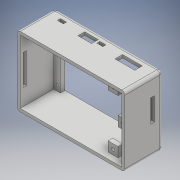
# Autodesk Inventor part: ttgofront
Saved by Autodesk Inventor 2017 (Build 210142000, 142)
## iProperties
Created: 2018-11-11
Part Number: ttgofront
Material: Generic
Document SubType Name: Modeling
Designer: simulator
Density: 1 g/cm^3
Appearance: Default
Author: simulator
Autodesk Inventor part; units mm, degrees
ref_plane "YZ Plane" through (0, 0, 0) normal (1, 0, 0) x (0, 1, 0)
ref_plane "XZ Plane" through (0, 0, 0) normal (0, 1, 0) x (-1, 0, 0)
ref_plane "XY Plane" through (0, 0, 0) normal (0, 0, 1) x (1, 0, 0)
sketch "Sketch1" plane through (0, 0, 0) normal (0, 1, 0) x (-1, 0, 0)
  line L0 (0, 21) -> (-67, 21)
  line L1 (-67, 21) -> (-67, -21)
  line L2 (-67, -21) -> (0, -21)
  line L3 (0, -21) -> (0, 21)
  line L4 (-4.5, 21) -> (-4.5, -21)
  line L5 (-60.5, 21) -> (-60.5, -21)
  line L6 (2, 23) -> (-69, 23)
  line L7 (-69, 23) -> (-69, -23)
  line L8 (-69, -23) -> (2, -23)
  line L9 (2, -23) -> (2, 23)
  line L10 (-32.322, -31.2235) -> (-36.822, -31.2235)
  line L11 (-36.822, -31.2235) -> (-36.822, -37.7235)
  line L12 (-36.822, -37.7235) -> (-32.322, -37.7235)
  line L13 (-32.322, -37.7235) -> (-32.322, -31.2235)
  line L14 (-32.322, -37.7235) -> (-36.822, -31.2235)
  line L15 (-67, -8.75) -> (-67, -15.25)
  line L16 (-67, 2.25) -> (-67, -4.25)
  line L17 (-67, 12.25) -> (-67, 5.75)
  line L18 (-66, -15.25) -> (-61.5, -15.25)
  line L19 (-61.5, -15.25) -> (-61.5, 14.25)
  line L20 (-61.5, 14.25) -> (-66, 14.25)
  line L21 (-66, 14.25) -> (-66, -15.25)
  point P0 (0, 0)
  point P1 (0, 0)
  point P2 (-2.5, -17.5)
  point P3 (-2.5, 18.5)
  point P4 (-63.5, 18.5)
  point P5 (-63.5, -17.5)
  point P6 (-34.572, -34.4735)
  dimension "d0" = 67
  dimension "d1" = 42
  dimension "d5" = 2.5
  dimension "d6" = 36
  dimension "d7" = 2.5
  dimension "d8" = 3.5
  dimension "d9" = 2.5
  dimension "d10" = 3.5
  dimension "d11" = 3.5
  dimension "d12" = 4.5
  dimension "d13" = 6.5
  dimension "d14" = 2
  dimension "d20" = 4.5
  dimension "d21" = 6.5
  dimension "d97" = 6.5
  dimension "d99" = 6.5
  dimension "d107" = 6.5
  dimension "d108" = 1
  dimension "d111" = 6.75
  dimension "d112" = 5.75
  dimension "d113" = 4.5
  constraints: 44 end point, 8 parallel, 6 perpendicular, 4 point on line, 3 horizontal, 2 midpoint, 1 coincident, 3 other
  measures "d0" distance of L2.end L1.end
  measures "d1" distance of L2.end L0.start
  measures "d5" distance from line of point (-2.5, -17.5) L3
  measures "d6" distance of point (-2.5, -17.5) point (-2.5, 18.5)
  measures "d7" distance from line of L0 point (-2.5, 18.5)
  measures "d8" distance from line of point (-63.5, 18.5) L1
  measures "d9" distance from line of L0 point (-63.5, 18.5)
  measures "d10" distance from line of point (-63.5, -17.5) L1
  measures "d11" distance from line of point (-63.5, -17.5) L2
  measures "d12" distance between parallel lines of L3 L4
  measures "d13" distance between parallel lines of L5 L1
  measures "d14" distance between parallel lines of L6 L0
  measures "d20" distance of L12.end L11.end
  measures "d21" distance of L11.end L10.end
  measures "d97" distance of L15.end L15.start
  measures "d99" distance of L16.end L16.start
  measures "d107" distance of L17.end L17.start
  measures "d108" distance from line of L18.start L1
  measures "d111" distance between parallel lines of L0 L20
  measures "d112" distance between parallel lines of L2 L18
  measures "d113" distance of L19.end L20.end
extrude "Extrusion1" add sketch "Sketch1" along normal blind 3 contours L3 L2 L4 L0 | L5 L2 L1 L0 | L9 L8 L7 L6 | L21 L20 L19 L18
sketch "Sketch2" plane through (0, 0, 0) normal (0, -1, 0) x (1, 0, 0)
  point P0 (0, 0)
  point P1 (2.5, 18.5)
  point P2 (2.5, -17.5)
  point P3 (63.5, -17.5)
  point P4 (63.5, 18.5)
hole "Hole1" at (2.5, 0, -17.5) at (2.5, 0, 18.5) at (63.5, 0, 18.5) at (63.5, 0, -17.5) direction (0, 1, 0) diameter 1.5 depth 2 tip angle 118
extrude "Extrusion2" add sketch "Sketch1" against normal blind 15 contours L9 L8 L7 L6
fillet "Fillet1" radius 2 8 edges at (-2, -6, 23) (-2, -6, -23) (69, -6, 23) (69, -6, -23) (33.5, 3, -23) (69, 3, 0) (33.5, 3, 23) (-2, 3, 0)
sketch "Sketch3" plane through (-2, -15, -21) normal (-1, 0, 0) x (0, 0, 1)
  line L0 (42, 15) -> (0, 15) projected
  line L1 (42, 16) -> (42, 0) projected
  point P0 (21, 15)
  point P1 (34.5, 7.5)
  dimension "d40" = 7.5
  dimension "d41" = 7.5
  measures "d40" distance from line of point (34.5, 7.5) L0
  measures "d41" distance from line of point (34.5, 7.5) L1
hole "Hole2" at (-2, -7.5, 13.5) direction (1, 0, 0) diameter 5.5 depth 5 tip angle 118
sketch "Sketch4" plane through (0, -15, 0) normal (0, -1, 0) x (1, 0, 0)
  arc A0 (67, -23) -> (69, -21) centre (67, -21) ccw projected
  line L0 (69, -21) -> (69, 21) projected
  arc A1 (69, 21) -> (67, 23) centre (67, 21) ccw projected
  line L1 (67, 23) -> (0, 23) projected
  arc A2 (0, 23) -> (-2, 21) centre (0, 21) ccw projected
  line L2 (-2, 21) -> (-2, -21) projected
  arc A3 (-2, -21) -> (0, -23) centre (0, -21) ccw projected
  line L3 (0, -23) -> (67, -23) projected
  line L4 (67, -21) -> (0, -21) projected
  line L5 (0, -21) -> (0, 21) projected
  line L6 (0, 21) -> (67, 21) projected
  line L7 (67, 21) -> (67, -21) projected
  line L8 (67, 21) -> (60.5, 21) projected
  line L9 (67, 21) -> (62, 21)
  line L10 (62, 21) -> (62, 16)
  line L11 (62, 16) -> (67, 16)
  line L12 (67, 16) -> (67, 21)
  line L13 (60.5, -21) -> (67, -21) projected
  line L14 (67, -21) -> (62, -21)
  line L15 (62, -21) -> (62, -16)
  line L16 (62, -16) -> (67, -16)
  line L17 (67, -16) -> (67, -21)
  line L18 (0, -21) -> (5, -21)
  line L19 (5, -21) -> (5, -16)
  line L20 (5, -16) -> (0, -16)
  line L21 (0, -16) -> (0, -21)
  line L22 (0, 21) -> (5, 21)
  line L23 (5, 21) -> (5, 16)
  line L24 (5, 16) -> (0, 16)
  line L25 (0, 16) -> (0, 21)
  point P0 (0, 0)
  dimension "d49" = 5
  dimension "d50" = 5
  dimension "d51" = 5
  dimension "d52" = 5
  dimension "d53" = 5
  dimension "d54" = 5
  dimension "d55" = 5
  dimension "d56" = 5
  constraints: 32 end point, 8 parallel, 4 horizontal, 4 perpendicular
  measures "d49" distance of L11.end L10.end
  measures "d50" distance of L10.end L9.end
  measures "d51" distance of L15.end L16.end
  measures "d52" distance of L14.end L15.end
  measures "d53" distance of L20.end L19.end
  measures "d54" distance of L19.end L18.end
  measures "d55" distance of L23.end L24.end
  measures "d56" distance of L22.end L23.end
sketch "Sketch6" plane through (69, 1, 21) normal (1, 0, 0) x (0, 0, -1)
  line L0 (42, 0) -> (42, -16) projected
  line L1 (0, 0) -> (42, 0) projected
  line L2 (0, -16) -> (0, 0) projected
  line L3 (42, -1) -> (0, -1) projected
  line L4 (25, -3.5) -> (10, -3.5)
  line L5 (10, -3.5) -> (10, -6)
  line L6 (10, -6) -> (25, -6)
  line L7 (25, -6) -> (25, -3.5)
  line L8 (42, -1) -> (42, -16) projected
  line L9 (0, -1) -> (0, -16) projected
  line L10 (42, -1) -> (0, -1) projected
  line L11 (0, -16) -> (42, -16) projected
  line L12 (42, -16) -> (0, -16) projected
  point P0 (21, -1)
  dimension "d68" = 15
  dimension "d69" = 2.5
  dimension "d70" = 10
  dimension "d71" = 2.5
  constraints: 8 end point, 2 parallel, 1 horizontal, 1 perpendicular
  measures "d68" distance of L6.end L5.end
  measures "d69" distance of L5.end L4.end
  measures "d70" distance between parallel lines of L5 L2
  measures "d71" distance between parallel lines of L3 L4
extrude "Extrusion5" cut sketch "Sketch6" against normal blind 10 contours L7 L6 L5 L4
sketch "Sketch7" plane through (0, 1, 23) normal (0, 0, 1) x (1, 0, 0)
  line L0 (67, 0) -> (67, 2) projected
  line L1 (67, 2) -> (60.5, 2) projected
  line L2 (60.5, 2) -> (4.5, 2) projected
  line L3 (4.5, 2) -> (0, 2) projected
  line L4 (0, 2) -> (0, 0) projected
  line L5 (0, 0) -> (67, 0) projected
  line L6 (67, 0) -> (67, -16) projected
  line L7 (0, 0) -> (67, 0) projected
  line L8 (0, -16) -> (0, 0) projected
  line L9 (-16.7799, -1) -> (83.7799, -1) projected
  line L10 (15.2278, 9.5342) -> (19.2278, 9.5342)
  line L11 (19.2278, 9.5342) -> (19.2278, 11.5342)
  line L12 (19.2278, 11.5342) -> (15.2278, 11.5342)
  line L13 (15.2278, 11.5342) -> (15.2278, 9.5342)
  line L14 (19.2278, 9.5342) -> (15.2278, 11.5342)
  line L15 (21.5, -6.5) -> (30.5, -6.5)
  line L16 (30.5, -6.5) -> (30.5, -2)
  line L17 (30.5, -2) -> (21.5, -2)
  line L18 (21.5, -2) -> (21.5, -6.5)
  line L19 (60, -2.5) -> (47, -2.5)
  line L20 (47, -2.5) -> (47, -7.5)
  line L21 (47, -7.5) -> (60, -7.5)
  line L22 (60, -7.5) -> (60, -2.5)
  line L23 (6, -4.5) -> (10, -4.5)
  line L24 (10, -4.5) -> (10, -2.5)
  line L25 (10, -2.5) -> (6, -2.5)
  line L26 (6, -2.5) -> (6, -4.5)
  line L27 (10, -4.5) -> (6, -2.5)
  line L28 (32, -4.5) -> (36, -4.5)
  line L29 (36, -4.5) -> (36, -2.5)
  line L30 (36, -2.5) -> (32, -2.5)
  line L31 (32, -2.5) -> (32, -4.5)
  line L32 (36, -4.5) -> (32, -2.5)
  line L33 (67, -16) -> (0, -16) projected
  point P0 (0, -1)
  point P1 (8, -3.5)
  point P2 (17.2278, 10.5342)
  point P3 (34, -3.5)
  point P4 (8, -3.5)
  point P5 (34, -3.5)
  dimension "d74" = 2.5
  dimension "d75" = 8
  dimension "d76" = 4
  dimension "d77" = 2
  dimension "d78" = 21.5
  dimension "d79" = 30.5
  dimension "d80" = 4.5
  dimension "d81" = 1
  dimension "d82" = 34
  dimension "d83" = 2.5
  dimension "d84" = 47
  dimension "d85" = 60
  dimension "d86" = 5
  dimension "d87" = 1.5
  dimension "d88" = 4
  dimension "d89" = 2
  dimension "d90" = 4
  dimension "d91" = 2
  constraints: 46 end point, 10 parallel, 5 horizontal, 5 perpendicular, 3 midpoint
  measures "d74" distance from line of point (8, -3.5) L9
  measures "d75" distance from line of point (8, -3.5) L8
  measures "d76" distance of L12.end L11.end
  measures "d77" distance of L11.end L10.end
  measures "d78" distance between parallel lines of L8 L18
  measures "d79" distance between parallel lines of L8 L16
  measures "d80" distance of L17.end L15.start
  measures "d81" distance between parallel lines of L17 L9
  measures "d82" distance from line of point (34, -3.5) L8
  measures "d83" distance from line of point (34, -3.5) L9
  measures "d84" distance between parallel lines of L20 L8
  measures "d85" distance between parallel lines of L8 L22
  measures "d86" distance of L19.end L20.end
  measures "d87" distance between parallel lines of L19 L9
  measures "d88" distance of L25.end L24.end
  measures "d89" distance of L24.end L23.end
  measures "d90" distance of L30.end L29.end
  measures "d91" distance of L29.end L28.end
extrude "Extrusion6" cut sketch "Sketch7" against normal blind 10 contours L18 L17 L16 L15 | L22 L21 L20 L19 | L26 L27 L23 | L27 L25 L24 | L31 L32 L28 | L32 L30 L29
extrude "Extrusion7" cut sketch "Sketch1" along normal through all contours L21 L20 L19 L18
sketch "Sketch8" plane through (0, -15, 0) normal (0, -1, 0) x (1, 0, 0)
  arc A0 (67, -23) -> (69, -21) centre (67, -21) ccw projected
  line L0 (69, -21) -> (69, 21) projected
  arc A1 (69, 21) -> (67, 23) centre (67, 21) ccw projected
  line L1 (67, 23) -> (0, 23) projected
  arc A2 (0, 23) -> (-2, 21) centre (0, 21) ccw projected
  line L2 (-2, 21) -> (-2, -21) projected
  arc A3 (-2, -21) -> (0, -23) centre (0, -21) ccw projected
  line L3 (0, -23) -> (67, -23) projected
  line L4 (67, -21) -> (0, -21) projected
  line L5 (0, -21) -> (0, 21) projected
  line L6 (0, 21) -> (67, 21) projected
  line L7 (67, 21) -> (67, -21) projected
  line L8 (67, 21) -> (60.5, 21)
  line L9 (60.5, 21) -> (60.5, 14.5)
  line L10 (67, 14.5) -> (67, 21)
  line L11 (67, -21) -> (67, 21) projected
  line L12 (60.5, -21) -> (60.5, -14.5)
  line L13 (67, -14.5) -> (67, -21)
  line L14 (67, 21) -> (69, 21) projected
  line L15 (54, 14.5) -> (60.5, 14.5)
  line L16 (60.5, 14.5) -> (60.5, 21)
  line L17 (60.5, 21) -> (54, 21)
  line L18 (54, 21) -> (54, 14.5)
  line L19 (54, -21) -> (60.5, -21)
  line L20 (60.5, -21) -> (60.5, -14.5)
  line L21 (60.5, -14.5) -> (54, -14.5)
  line L22 (54, -14.5) -> (54, -21)
  line L23 (54, 21) -> (60.5, 14.5)
  line L24 (54, -21) -> (60.5, -14.5)
  line L25 (60.5, -3.25) -> (67, -3.25)
  line L26 (67, -3.25) -> (67, 3.25)
  line L27 (67, 3.25) -> (60.5, 3.25)
  line L28 (60.5, 3.25) -> (60.5, -3.25)
  line L29 (60.5, 3.25) -> (67, -3.25)
  line L30 (67, 14.5) -> (67, -14.5)
  point P0 (0, 0)
  point P1 (67, 0)
  point P2 (57.25, 17.75)
  point P3 (63.75, 0)
  point P4 (57.25, -17.75)
  dimension "d115" = 6.5
  dimension "d117" = 6.5
  dimension "d157" = 6.5
  dimension "d159" = 6.5
  dimension "d162" = 6.5
  dimension "d163" = 6.5
  dimension "d164" = 6.5
  constraints: 42 end point, 8 parallel, 5 midpoint, 4 horizontal, 4 perpendicular, 1 collinear, 1 point on line
  measures "d115" distance of L9.end L8.end
  measures "d117" distance of L12.start L12.end
  measures "d157" distance of L17.end L16.end
  measures "d159" distance of L21.end L20.end
  measures "d162" distance of L26.end L25.end
  measures "d163" distance between parallel lines of L16 L10
  measures "d164" distance between parallel lines of L11 L20
extrude "Extrusion8" add sketch "Sketch8" along normal blind 3 contours L3 A3 L2 A2 L1 A1 L0 A0 | L4 L24 L12 | L22 L21 L24 | L29 L27 L7 | L25 L28 L29 | L23 L15 L18 | L6 L9 L23
sketch "Sketch9" plane through (0, -18, 0) normal (0, -1, 0) x (1, 0, 0)
  line L0 (67, -21) -> (60.5, -21) projected
  line L1 (0, -21) -> (0, 21) projected
  line L2 (0, 21) -> (54, 21) projected
  line L3 (67, 21) -> (67, 3.25) projected
  arc A0 (67, -23) -> (69, -21) centre (67, -21) ccw projected
  line L4 (69, -21) -> (69, 21) projected
  arc A1 (69, 21) -> (67, 23) centre (67, 21) ccw projected
  line L5 (67, 23) -> (0, 23) projected
  arc A2 (0, 23) -> (-2, 21) centre (0, 21) ccw projected
  line L6 (-2, 21) -> (-2, -21) projected
  arc A3 (-2, -21) -> (0, -23) centre (0, -21) ccw projected
  line L7 (0, -23) -> (67, -23) projected
  line L8 (69, -21) -> (67, -21) projected
  line L9 (67, -21) -> (60.5, -14.5)
  line L10 (67, 21) -> (69, 21) projected
  line L11 (67, 21) -> (60.5, 14.5)
  line L12 (60.5, -21) -> (60.5, -14.5) projected
  line L13 (60.5, -14.5) -> (54, -14.5) projected
  line L14 (54, -14.5) -> (54, -21) projected
  line L15 (54, -21) -> (0, -21) projected
  line L16 (54, 21) -> (54, 14.5) projected
  line L17 (54, 14.5) -> (60.5, 14.5) projected
  line L18 (60.5, 14.5) -> (60.5, 21) projected
  line L19 (60.5, 21) -> (67, 21) projected
  line L20 (67, 3.25) -> (60.5, 3.25) projected
  line L21 (60.5, 3.25) -> (60.5, -3.25) projected
  line L22 (60.5, -3.25) -> (67, -3.25) projected
  line L23 (67, -3.25) -> (67, -21) projected
  point P0 (0, 0)
  point P1 (63.75, -17.75)
  point P2 (63.75, 17.75)
  constraints: 4 end point, 2 midpoint, 1 perpendicular
sketch "Sketch10" plane through (0, -18, 0) normal (0, -1, 0) x (1, 0, 0)
  line L0 (0, 16.25) -> (-2, 16.25) projected
  line L1 (67, -21) -> (60.5, -21) projected
  line L2 (0, -21) -> (0, 21) projected
  line L3 (0, 21) -> (54, 21) projected
  line L4 (67, 21) -> (67, 3.25) projected
  arc A0 (67, -23) -> (69, -21) centre (67, -21) ccw projected
  line L5 (69, -21) -> (69, 21) projected
  arc A1 (69, 21) -> (67, 23) centre (67, 21) ccw projected
  line L6 (67, 23) -> (0, 23) projected
  arc A2 (0, 23) -> (-2, 21) centre (0, 21) ccw projected
  line L7 (-2, 21) -> (-2, -21) projected
  arc A3 (-2, -21) -> (0, -23) centre (0, -21) ccw projected
  line L8 (0, -23) -> (67, -23) projected
  line L9 (-2, -10) -> (0, -10)
  line L10 (0, -10) -> (0, 10)
  line L11 (0, 10) -> (-2, 10)
  line L12 (-2, 10) -> (-2, -10)
  line L13 (0, -21) -> (4.5, -21) projected
  line L14 (67, 21) -> (0, 21)
  line L15 (0, 21) -> (0, -21)
  line L16 (0, -21) -> (67, -21)
  line L17 (67, -21) -> (67, 21)
  line L18 (60.5, -21) -> (60.5, -14.5) projected
  line L19 (60.5, -14.5) -> (54, -14.5) projected
  line L20 (54, -14.5) -> (54, -21) projected
  line L21 (54, -21) -> (0, -21) projected
  line L22 (54, 21) -> (54, 14.5) projected
  line L23 (54, 14.5) -> (60.5, 14.5) projected
  line L24 (60.5, 14.5) -> (60.5, 21) projected
  line L25 (60.5, 21) -> (67, 21) projected
  line L26 (67, 3.25) -> (60.5, 3.25) projected
  line L27 (60.5, 3.25) -> (60.5, -3.25) projected
  line L28 (60.5, -3.25) -> (67, -3.25) projected
  line L29 (67, -3.25) -> (67, -21) projected
  point P0 (0, 0)
  dimension "d127" = 10
  dimension "d128" = 10
  constraints: 16 end point, 4 parallel, 2 horizontal, 2 perpendicular, 2 point on line
  measures "d127" distance from line of point (0, 0) L11
  measures "d128" distance from line of point (0, 0) L9
extrude "Extrusion9" add sketch "Sketch10" along normal blind 2 contours L2 L11 L7 L0 | L0 L7 A2 L6 A1 L5 A0 L8 A3 L9 L2 L13 L16 L1 L17 L4 L14 L3
sketch "Sketch11" plane through (0, -20, 0) normal (0, -1, 0) x (1, 0, 0)
  line L0 (0, -21) -> (0, -10) projected
  line L1 (0, -10) -> (-2, -10) projected
  line L2 (-2, -10) -> (-2, -21) projected
  arc A0 (-2, -21) -> (0, -23) centre (0, -21) ccw projected
  line L3 (0, -23) -> (67, -23) projected
  arc A1 (67, -23) -> (69, -21) centre (67, -21) ccw projected
  line L4 (69, -21) -> (69, 21) projected
  arc A2 (69, 21) -> (67, 23) centre (67, 21) ccw projected
  line L5 (67, 23) -> (0, 23) projected
  arc A3 (0, 23) -> (-2, 21) centre (0, 21) ccw projected
  line L6 (-2, 21) -> (-2, 10) projected
  line L7 (-2, 10) -> (0, 10) projected
  line L8 (0, 10) -> (0, 21) projected
  line L9 (0, 21) -> (67, 21) projected
  line L10 (67, 21) -> (67, -21) projected
  line L11 (67, -21) -> (0, -21) projected
  line L12 (-2, -10) -> (0, -10) projected
  line L13 (0, -10) -> (0, 10) projected
  line L14 (0, 10) -> (-2, 10) projected
  line L15 (-2, 10) -> (-2, -10) projected
  point P0 (0, 0)
extrude "Extrusion10" add sketch "Sketch11" along normal blind 2 contours L11 L10 L9 L8 L7 L6 A3 L5 A2 L4 A1 L3 A0 L2 L1 L0 | L1 L15 L7 L13
sketch "Sketch13" plane through (0, 3, 0) normal (0, 1, 0) x (1, 0, 0)
  line L0 (66, 15.25) -> (66, -14.25) projected
  line L1 (66, -14.25) -> (61.5, -14.25) projected
  line L2 (61.5, -14.25) -> (61.5, 15.25) projected
  line L3 (61.5, 15.25) -> (66, 15.25) projected
  line L4 (67, -21) -> (60.5, -21) projected
  line L5 (67, 21) -> (67, -21) projected
  line L6 (60.5, 21) -> (67, 21) projected
  line L7 (60.5, 21) -> (60.5, -21) projected
  line L8 (66, -14.25) -> (66, 15.25) projected
  line L9 (66, -13.25) -> (62, -13.25)
  line L10 (62, -13.25) -> (62, -6.75)
  line L11 (62, -6.75) -> (66, -6.75)
  line L12 (66, -6.75) -> (66, -13.25)
  line L13 (66, 14.25) -> (62, 14.25)
  line L14 (62, 14.25) -> (62, 7.75)
  line L15 (62, 7.75) -> (66, 7.75)
  line L16 (66, 7.75) -> (66, 14.25)
  line L17 (66, 3.75) -> (62, 3.75)
  line L18 (62, 3.75) -> (62, -2.75)
  line L19 (62, -2.75) -> (66, -2.75)
  line L20 (66, -2.75) -> (66, 3.75)
  line L21 (61.5, -14.25) -> (66, -14.25) projected
  line L22 (66, -14.25) -> (66, 15.25)
  point P0 (0, 0)
  point P1 (66, 0.5)
  dimension "d147" = 4
  dimension "d148" = 6.5
  dimension "d149" = 4
  dimension "d150" = 6.5
  dimension "d151" = 4
  dimension "d152" = 6.5
  dimension "d153" = 1
  dimension "d154" = 1
  constraints: 26 end point, 7 parallel, 3 horizontal, 3 perpendicular, 3 point on line, 2 midpoint
  measures "d147" distance of L10.end L11.end
  measures "d148" distance of L9.end L10.end
  measures "d149" distance of L15.end L14.end
  measures "d150" distance of L14.end L13.end
  measures "d151" distance of L19.end L18.end
  measures "d152" distance of L18.end L17.end
  measures "d153" distance between parallel lines of L1 L9
  measures "d154" distance between parallel lines of L3 L13
extrude "Extrusion12" add sketch "Sketch13" against normal blind 0.5 contours L0 L15 L14 L13 | L0 L19 L18 L17 | L9 L10 L11 L0
hole "Hole5" at (57.25, -15, 17.75) at (63.75, -15, 0) at (57.25, -15, -17.75) direction (0, -1, 0) diameter 2 depth 8 tip angle 118
body "Solid1"
